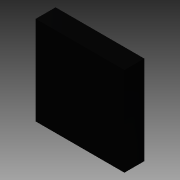
# Autodesk Inventor part: MPU6050
Saved by Autodesk Inventor 2013 (Build 170138000, 138)
## iProperties
Created: 2015-07-01
Part Number: MPU6050
Material: Ogólny
Document SubType Name: Modeling
Designer: terg
Density: 1 g/cm^3
Author: terg
Autodesk Inventor part; units mm, degrees
ref_plane "YZ Plane" through (0, 0, 0) normal (1, 0, 0) x (0, 1, 0)
ref_plane "XZ Plane" through (0, 0, 0) normal (0, 1, 0) x (-1, 0, 0)
ref_plane "XY Plane" through (0, 0, 0) normal (0, 0, 1) x (1, 0, 0)
sketch "Szkic1" plane through (0, 0, 0) normal (0, 1, 0) x (-1, 0, 0)
  line L0 (0, 0) -> (4, 0)
  line L1 (4, 0) -> (4, 4)
  line L2 (4, 4) -> (0, 4)
  line L3 (0, 4) -> (0, 0)
  dimension "d0" = 4
  dimension "d1" = 4
  constraints: 8 end point, 2 parallel, 1 horizontal, 1 perpendicular
  measures "d0" distance of L2.end L1.end
  measures "d1" distance of L1.end L0.end
extrude "Wyciągnięcie proste1" add sketch "Szkic1" along normal blind 0.9
sketch "Szkic2" plane through (0, 0.9, 0) normal (0, 1, 0) x (1, 0, 0)
  line L0 (0, 0) -> (-4, 0) projected
  line L1 (-4, 0) -> (-4, -4) projected
  point P0 (-3.6, -0.4)
  dimension "d4" = 0.4
  dimension "d5" = 0.4
  measures "d4" distance from line of point (-3.6, -0.4) L1
  measures "d5" distance from line of L0 point (-3.6, -0.4)
hole "Otwór1" at (-3.6, 0.9, 0.4) direction (0, -1, 0) diameter 0.3 depth 0.1
